Autodesk Fusion 360 part; units mm, degrees
(part 2 of 2)
extrude "Extrusion20" cut sketch "Esquisse29" against normal blind 2 contours L0 L1 L2 L3 | S0 L4 L5 L6 S1 S2 S3 S4 L7 L8 L9 L10 L11 S5 S6 S7 L12 | S8 S9 L13 S10 S11 S12 S13 S14 S15 S16 S17 S18 S19 S20 S21 S22 S23 L14 S24 S25 S26 S27 S28 S29 S30 S31 S32 S33 S34 S35 S36 | L15 S37 S38 S39 L16 S40 S41 S42 S43 S44 S45 S46 S47 S48 S49 S50 S51 S52 L17 | L18 L19 L20 L21 | S57 L23 L24 S58 S59 L25 L26 L27 L28 L29 S60 L30 | L31 S61 S62 S63 L32 S64 S65 S66 S67 S68 S69 S70 S71 S72 S73 S74 S75 S76 L33 | L35 L36 S81 S82 L37 L38 L39 L40 L41 L42 L43 L44 L45 L46 L47 S83 S84 L48 | S85 S86 S87 S88 S89 S90 S91 S92 S93 S94 S95 S96 L49 | S105 L51 L52 L53 S106 S107 S108 S109 L54 L55 L56 L57 L58 S110 S111 S112 L59 | S113 S114 S115 S116 L60 L61 L62 L63 L64 S117 S118 S119 S120 S121 S122 L65 | L67 S131 S132 S133 L68 S134 S135 S136 S137 S138 S139 S140 S141 S142 S143 S144 S145 S146 L69 | S151 S152 L71 S153 S154 S155 S156 S157 S158 S159 S160 S161 S162 S163 S164 S165 S166 L72 S167 S168 S169 S170 S171 S172 S173 S174 S175 S176 S177 S178 S179 | S180 S181 L73 S182 S183 S184 S185 S186 S187 S188 S189 S190 S191 S192 S193 S194 S195 L74 S196 S197 S198 S199 S200 S201 S202 S203 S204 S205 S206 S207 S208 | S209 S210 S211 S212 S213 S214 S215 S216 | L75 L76 L77 L78 | S217 L79 L80 L81 S218 S219 S220 S221 L82 L83 L84 L85 L86 S222 S223 S224 L87 | S225 S226 S227 S228 S229 S230 S231 S232 | L88 L89 L90 L91 | S233 S234 S235 S236 L92 S237 S238 S239 S240 S241 S242 L93 S243 S244 S245 S246 S247 S248 | S249 S250 S251 S252 S253 S254 S255 S256 | L94 L95 L96 L97 bodies 5
sketch "Esquisse36" plane through (200, 0, 0) normal (1, 0, 0) x (0, 0, 1)
  spline S0 degree 3 poles (-13.1557, -805.3703) (-12.8926, -805.1852) (1.1077, -795.064) (1.1914, -794.9998) knots 0 0 0 0 1 1 1 1
  line L0 (1.1914, -794.9998) -> (1.299, -794.9167)
  line L1 (1.299, -794.9167) -> (8.4498, -800.0868)
  spline S1 degree 3 poles (8.4498, -800.0868) (12.3816, -802.9297) (15.6437, -805.2909) (15.6987, -805.3325) knots 3 3 3 3 4 4 4 4
  line L2 (15.6987, -805.3325) -> (15.8015, -805.41)
  line L3 (15.8015, -805.41) -> (15.8015, -800.9595)
  line L4 (15.8015, -800.9595) -> (15.8015, -796.5072)
  line L5 (15.8015, -796.5072) -> (8.5526, -791.2653)
  line L6 (8.5526, -791.2653) -> (1.3038, -786.0214)
  line L7 (1.3038, -786.0214) -> (1.1435, -786.1367)
  spline S2 degree 3 poles (1.1435, -786.1367) (1.0574, -786.2009) (-2.2071, -788.5602) (-6.1101, -791.3824) knots 10 10 10 10 11 11 11 11
  line L8 (-6.1101, -791.3824) -> (-13.2083, -796.5147)
  line L9 (-13.2083, -796.5147) -> (-13.2083, -800.9614)
  line L10 (-13.2083, -800.9614) -> (-13.2083, -805.4081)
  line L11 (-13.2083, -805.4081) -> (-13.1557, -805.3703)
extrude "Extrusion24" cut sketch "Esquisse36" against normal blind 2 bodies 5
copy_body "Copier/Coller des corps3" bodies 9 makes body 13
move_body "Déplacer3" bodies 13 to x (1, 0, 0) y (0, 1, 0) z (0, 0, 1) at (0, -600, 0)
